Autodesk Fusion 360 part; units mm, degrees
(part 2 of 2)
sketch "Sketch13" plane through (-99.5, 0, 0) normal (-1, 0, 0) x (0, -1, 0) in component "backing-frame"
  line L0 (63, -5) -> (-66, -5)
  line L1 (-66, -5) -> (-66, -28.3)
  line L2 (63, -28.3) -> (63, -5)
  line L3 (-66, -10) -> (63, -10) construction
  line L4 (-58.5, -10) -> (-55.9997, -74.9519) construction
  line L5 (-58.5, -10) -> (2.1654, -10) construction
  circle A0 centre (-58.5, -10) radius 5 construction
  circle A1 centre (-58.5, -10) radius 10 construction
  line L6 (-68.5, -5) -> (-66, -5) construction
  line L7 (-68.5, -5) -> (-68.5, -28.3) construction
  line L8 (-66, -28.3) -> (-66, -5) construction
  line L9 (-55.9997, -74.9519) -> (-68.5, -28.3) construction
  line L10 (-66, -28.3) -> (63, -28.3)
  line L11 (-68.5, -28.3) -> (-66, -28.3)
  point P0 (-57.9107, -25.3084)
  dimension "d215" = 5
  dimension "d217" = 10
  dimension "d218" = 20
  dimension "d220" = 15
  dimension "d221" = 65
  constraint coincident L1 L3.start
  constraint coincident L2 L3.end
  constraint perpendicular L2 L3
  constraint horizontal L5
  constraint coincident L3 L4.start
  constraint coincident L4.start L5.start
  constraint concentric A0 A1
  constraint tangent A1 L7
  constraint coincident L7.end L9.end
  constraint coincident L4 P0
  measures "d215" distance of L0 L3
  measures "d217" diameter of A0
  measures "d218" diameter of A1
  measures "d220" angle of L7 L9
  measures "d221" distance of L4.start L4.end
sketch "Sketch1 (7)" plane through (0, 0, 0.5) normal (0, 0, 1) x (-1, 0, 0) in component "tape"
  line L0 (-86, -56) -> (86, -56)
  line L1 (86, -56) -> (86, 56)
  line L2 (86, 56) -> (-86, 56)
  line L3 (-86, 56) -> (-86, -56)
  line L4 (68, -38) -> (-68, -38)
  line L5 (-68, -38) -> (-68, 38)
  line L6 (-68, 38) -> (68, 38)
  line L7 (68, 38) -> (68, -38)
  line L8 (86, 56) -> (68, 56)
  line L9 (68, 56) -> (68, -56)
  line L10 (68, -56) -> (86, -56)
  line L11 (86, -56) -> (86, 56)
  line L12 (-86, 56) -> (-68, 56)
  line L13 (-68, 56) -> (-68, -56)
  line L14 (-68, -56) -> (-86, -56)
  line L15 (-86, -56) -> (-86, 56)
  line L16 (68, 38) -> (-68, 38)
  line L17 (-68, 38) -> (-68, 56)
  line L18 (-68, 56) -> (68, 56)
  line L19 (68, 56) -> (68, 38)
  line L20 (-68, -56) -> (68, -56)
  line L21 (68, -56) -> (68, -38)
  line L22 (68, -38) -> (-68, -38)
  line L23 (-68, -38) -> (-68, -56)
  constraint horizontal L8
  constraint vertical L9
  constraint horizontal L10
  constraint vertical L11
  constraint coincident L0 L9.end
  constraint coincident L1.end L2.start
  constraint horizontal L12
  constraint vertical L13
  constraint horizontal L14
  constraint vertical L15
  constraint coincident L0 L13.end
  constraint coincident L2.end L3.start
  constraint horizontal L16
  constraint vertical L17
  constraint horizontal L18
  constraint vertical L19
  constraint coincident L6.end L7.start
  constraint horizontal L20
  constraint vertical L21
  constraint horizontal L22
  constraint vertical L23
  constraint coincident L4.start L7.end
  constraint coincident L9 L4.start
  constraint coincident L4.end L13
extrude "Extrude1'''" add sketch "Sketch1 (7)" along normal blind 2 separate body contours L0 L2 L3 L5 L12 L13 L14 L15 L17 L23 | L0 L4 L9 L13 L20 L21 L22 L23 | L0 L1 L2 L7 L8 L9 L10 L11 L19 L21 | L2 L6 L9 L13 L16 L17 L18 L19 makes body 7 in component "tape"
sketch "Sketch1 (8)" plane through (0, 0, 2.5) normal (0, 0, 1) x (-1, 0, 0) in component "display"
  line L0 (-68, 38) -> (68, 38)
  line L1 (68, -38) -> (-68, -38)
  line L2 (-68, -38) -> (-68, 38)
  line L3 (-86, -56) -> (86, -56)
  line L4 (86, -56) -> (86, 56)
  line L5 (86, 56) -> (-86, 56)
  line L6 (-86, 56) -> (-86, -56)
  line L7 (86, -56) -> (-86, -56)
  line L8 (-86, -56) -> (-86, 56)
  line L9 (-86, 56) -> (86, 56)
  line L10 (86, 56) -> (86, -56)
  line L11 (68, 38) -> (68, -38)
  constraint horizontal L7
  constraint vertical L8
  constraint horizontal L9
  constraint vertical L10
  constraint coincident L5.end L6.start
  constraint coincident L3.end L4.start
extrude "Extrude1''''" add sketch "Sketch1 (8)" along normal blind 1 separate body contours L0 L1 L2 L11 | L3 L4 L5 L6 L7 L8 L9 L10 makes body 8 in component "display"
component "display-frame" placed x (1, 0, 0) y (0, 1, 0) z (0, 0, 1) at (0, 0, 0)
component "controller-frame" placed x (1, 0, 0) y (0, 1, 0) z (0, 0, 1) at (0, 0, 0)
component "backing-frame" placed x (1, 0, 0) y (0, 1, 0) z (0, 0, 1) at (0, 0, 0)
component "glass-frame" placed x (1, 0, 0) y (0, 1, 0) z (0, 0, 1) at (0, 0, 0)
component "backing" placed x (1, 0, 0) y (0, 1, 0) z (0, 0, 1) at (0, 0, 0)
component "tape" placed x (1, 0, 0) y (0, 1, 0) z (0, 0, 1) at (0, 0, 0)
component "display" placed x (1, 0, 0) y (0, 1, 0) z (0, 0, 1) at (0, 0, 0)
component "bolt-test" placed x (1, 0, 0) y (0, 1, 0) z (0, 0, 1) at (0, 0, 0)
equation "d2 = ( 70 * 2 ) * 1 mm + 30 mm + 2 mm"
equation "d4 = ( 30 / 2 ) * 1 mm"
equation "d23 = 3.50 mm - 1 mm"
equation "d118 = d117 / 2"
equation "d119 = d118"
equation "d120 = d118"
equation "d121 = d118"
equation "d124 = d123 / 3"
equation "d125 = d124"
equation "d140 = 3 mm + 2 mm"
equation "d162 = d163"
equation "d164 = d163"
equation "d166 = d163"
equation "d167 = d163"
equation "d193 = -3.50 mm + 2.75 mm"
equation "d195 = 20 mm - 6.2 mm"
equation "d218 = d217 + 5 * 2 mm"
equation "d220 = 90 deg - 75 deg"
equation "d234 = 17 mm - d142 / 2 - d140 / 2"
equation "d235 = 41 mm - d141"
equation "d243 = d242 * 2 + 5 mm"
equation "d247 = 3.00 mm + 3.5 mm"
equation "d254 = d253 + 10 mm"
equation "d256 = d255 / 3"
equation "d259 = -20.30 mm + 5 mm"
